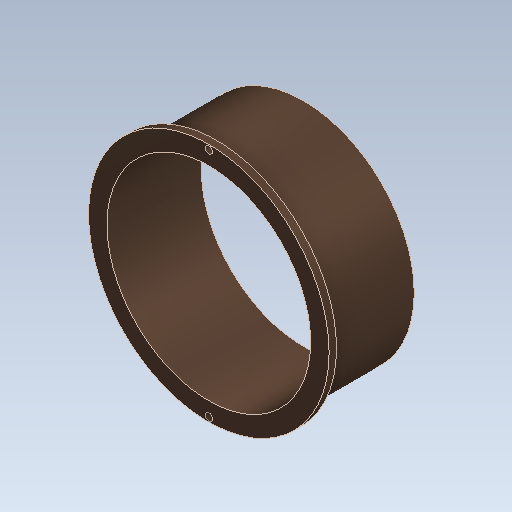
# Autodesk Inventor part: Втулка под палец_CPY
Saved by Autodesk Inventor 2021 (Build 250183000, 183)
## iProperties
Created: 2020-11-30
Part Number: Втулка под палец_CPY
Material: Бронза, литейная
Document SubType Name: Modeling
Designer: Тимоха
Mass: 901.964 g
Surface Area: 452.892 cm^2
Volume: 101.687 cm^3
Density: 8.87 g/cm^3
Appearance: Бронза - сатинированная
Author: Тимоха
Autodesk Inventor part; units mm, degrees
ref_plane "YZ Plane" through (0, 0, 0) normal (1, 0, 0) x (0, 1, 0)
ref_plane "XZ Plane" through (0, 0, 0) normal (0, 1, 0) x (-1, 0, 0)
ref_plane "XY Plane" through (0, 0, 0) normal (0, 0, 1) x (1, 0, 0)
sketch "Эскиз1" plane through (0, 0, 0) normal (0, 0, 1) x (1, 0, 0)
  circle A0 centre (0, 0) radius 60
  circle A1 centre (0, 0) radius 55
  dimension "d0" = 120
  dimension "d1" = 110
  constraints: 2 centre point, 2 coincident
  measures "d0" diameter of A0
  measures "d1" diameter of A1
extrude "Выдавливание1" add sketch "Эскиз1" along normal blind 51
sketch "Эскиз2" plane through (0, 0, 51) normal (0, 0, 1) x (1, 0, 0)
  circle A0 centre (0, 0) radius 60 projected
  circle A1 centre (0, 0) radius 65
  constraints: 1 centre point, 1 coincident
extrude "Выдавливание2" add sketch "Эскиз2" against normal blind 4
sketch "Эскиз3" plane through (0, 0, 51) normal (0, 0, 1) x (1, 0, 0)
  circle A0 centre (0, 0) radius 55 projected
  line L0 (0, 55) -> (0, 62.5)
  dimension "d6" = 7.5
  constraints: 2 end point, 1 vertical, 1 vertical alignment, 1 other
  measures "d6" distance of L0.start L0.end
hole "Отверстие1" at (0, 62.5, 51) direction (0, 0, -1) diameter 4 depth 15 tip angle 118
mirror "Зеркальное отражение1" about plane through (0, 0, 0) normal (0, 1, 0) of "Отверстие1"
